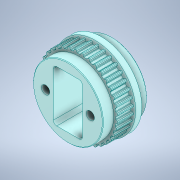
# Autodesk Inventor part: transmission_pulley_at3_t30_output
Saved by Autodesk Inventor 2022.2 (Build 262287000, 287)
## iProperties
Created: 2019-07-05
Part Number: transmission_pulley_at3_t30_output
Material: solidworks materials|PMMA
Document SubType Name: Modeling
Designer: Jochen
Density: 1.19 g/cm^3
Appearance: 192,255,255
Sending System: SolidWorks 2017
Last Author: Felix
Last Saved: 2021-02-23
Author: Jochen
Autodesk Inventor part; units mm, degrees
ref_plane "YZ Plane" through (0, 0, 0) normal (1, 0, 0) x (0, 1, 0)
ref_plane "XZ Plane" through (0, 0, 0) normal (0, 1, 0) x (-1, 0, 0)
feature "Fase1" [suppressed]
ref_plane "Work Plane1" through (0, 0, 20) normal (0, 0, 1) x (1, 0, 0)
sketch "Sketch1" plane through (0, 0, 20) normal (0, 0, 1) x (1, 0, 0)
  line L0 (-20.3, 0) -> (20.3, 0) construction
  line L1 (0, -20.3) -> (0, 20.3) construction
  line L2 (-4, -9) -> (4, -9)
  line L3 (5, -8) -> (5, 8) construction
  line L4 (4, 9) -> (-4, 9) construction
  line L5 (-5, 8) -> (-5, -8) construction
  line L6 (-5, -9) -> (5, 9) construction
  line L7 (5, -9) -> (-5, 9) construction
  circle A0 centre (0, 0) radius 12.5
  circle A1 centre (8, 0) radius 1.5
  circle A2 centre (-8, 0) radius 1.5
  arc A3 (-3.1617, 13.4663) -> (-3.482, 13.5848) centre (-3.4075, 13.2942) ccw
  arc A4 (-3.482, 13.5848) -> (-3.7769, 13.5058) centre (0, 0) ccw
  arc A5 (-3.7769, 13.5058) -> (-3.995, 13.243) centre (-3.6961, 13.2169) ccw
  line L8 (-3.995, 13.243) -> (-4.0355, 12.7799)
  arc A6 (-4.1663, 12.6094) -> (-4.0355, 12.7799) centre (-4.2348, 12.7973) ccw
  line L9 (-4.1663, 12.6094) -> (-4.9136, 12.3374)
  arc A7 (-5.1234, 12.384) -> (-4.9136, 12.3374) centre (-4.982, 12.5254) ccw
  line L10 (-5.1234, 12.384) -> (-5.4521, 12.7127)
  arc A8 (-5.4521, 12.7127) -> (-5.788, 12.7738) centre (-5.6642, 12.5005) ccw
  arc A9 (-5.788, 12.7738) -> (-6.0648, 12.6447) centre (0, 0) ccw
  arc A10 (-6.0648, 12.6447) -> (-6.2339, 12.3481) centre (-5.9351, 12.3742) ccw
  line L11 (-6.2339, 12.3481) -> (-6.1934, 11.885)
  arc A11 (-6.2927, 11.6944) -> (-6.1934, 11.885) centre (-6.3927, 11.8676) ccw
  line L12 (-6.2927, 11.6944) -> (-6.9813, 11.2968)
  arc A12 (-7.196, 11.3062) -> (-6.9813, 11.2968) centre (-7.0813, 11.47) ccw
  line L13 (-7.196, 11.3062) -> (-7.5768, 11.5728)
  arc A13 (-7.5768, 11.5728) -> (-7.9183, 11.5746) centre (-7.7489, 11.327) ccw
  arc A14 (-7.9183, 11.5746) -> (-8.1684, 11.3995) centre (0, 0) ccw
  arc A15 (-8.1684, 11.3995) -> (-8.2834, 11.078) centre (-7.9937, 11.1556) ccw
  line L14 (-8.2834, 11.078) -> (-8.1631, 10.629)
  arc A16 (-8.2278, 10.424) -> (-8.1631, 10.629) centre (-8.3563, 10.5772) ccw
  line L15 (-8.2278, 10.424) -> (-8.8369, 9.9129)
  arc A17 (-9.05, 9.8848) -> (-8.8369, 9.9129) centre (-8.9655, 10.0661) ccw
  line L16 (-9.05, 9.8848) -> (-9.4713, 10.0813)
  arc A18 (-9.4713, 10.0813) -> (-9.8079, 10.0238) centre (-9.5981, 9.8094) ccw
  arc A19 (-9.8079, 10.0238) -> (-10.0238, 9.8079) centre (0, 0) ccw
  arc A20 (-10.0238, 9.8079) -> (-10.0813, 9.4713) centre (-9.8094, 9.5981) ccw
  line L17 (-10.0813, 9.4713) -> (-9.8848, 9.05)
  arc A21 (-9.9129, 8.8369) -> (-9.8848, 9.05) centre (-10.0661, 8.9655) ccw
  line L18 (-9.9129, 8.8369) -> (-10.424, 8.2278)
  arc A22 (-10.629, 8.1631) -> (-10.424, 8.2278) centre (-10.5772, 8.3563) ccw
  line L19 (-10.629, 8.1631) -> (-11.078, 8.2834)
  arc A23 (-11.078, 8.2834) -> (-11.3995, 8.1684) centre (-11.1556, 7.9937) ccw
  arc A24 (-11.3995, 8.1684) -> (-11.5746, 7.9183) centre (0, 0) ccw
  arc A25 (-11.5746, 7.9183) -> (-11.5728, 7.5768) centre (-11.327, 7.7489) ccw
  line L20 (-11.5728, 7.5768) -> (-11.3062, 7.196)
  arc A26 (-11.2968, 6.9813) -> (-11.3062, 7.196) centre (-11.47, 7.0813) ccw
  line L21 (-11.2968, 6.9813) -> (-11.6944, 6.2927)
  arc A27 (-11.885, 6.1934) -> (-11.6944, 6.2927) centre (-11.8676, 6.3927) ccw
  line L22 (-11.885, 6.1934) -> (-12.3481, 6.2339)
  arc A28 (-12.3481, 6.2339) -> (-12.6447, 6.0648) centre (-12.3742, 5.9351) ccw
  arc A29 (-12.6447, 6.0648) -> (-12.7738, 5.788) centre (0, 0) ccw
  arc A30 (-12.7738, 5.788) -> (-12.7127, 5.4521) centre (-12.5005, 5.6642) ccw
  line L23 (-12.7127, 5.4521) -> (-12.384, 5.1234)
  arc A31 (-12.3374, 4.9136) -> (-12.384, 5.1234) centre (-12.5254, 4.982) ccw
  line L24 (-12.3374, 4.9136) -> (-12.6094, 4.1663)
  arc A32 (-12.7799, 4.0355) -> (-12.6094, 4.1663) centre (-12.7973, 4.2348) ccw
  line L25 (-12.7799, 4.0355) -> (-13.243, 3.995)
  arc A33 (-13.243, 3.995) -> (-13.5058, 3.7769) centre (-13.2169, 3.6961) ccw
  arc A34 (-13.5058, 3.7769) -> (-13.5848, 3.482) centre (0, 0) ccw
  arc A35 (-13.5848, 3.482) -> (-13.4663, 3.1617) centre (-13.2942, 3.4075) ccw
  line L26 (-13.4663, 3.1617) -> (-13.0855, 2.8951)
  arc A36 (-13.0032, 2.6965) -> (-13.0855, 2.8951) centre (-13.2002, 2.7313) ccw
  line L27 (-13.0032, 2.6965) -> (-13.1413, 1.9135)
  arc A37 (-13.2865, 1.755) -> (-13.1413, 1.9135) centre (-13.3383, 1.9482) ccw
  line L28 (-13.2865, 1.755) -> (-13.7355, 1.6347)
  arc A38 (-13.7355, 1.6347) -> (-13.9564, 1.3743) centre (-13.6579, 1.3449) ccw
  arc A39 (-13.9564, 1.3743) -> (-13.9831, 1.0701) centre (0, 0) ccw
  arc A40 (-13.9831, 1.0701) -> (-13.8107, 0.7753) centre (-13.6839, 1.0472) ccw
  line L29 (-13.8107, 0.7753) -> (-13.3894, 0.5788)
  arc A41 (-13.2739, 0.3976) -> (-13.3894, 0.5788) centre (-13.4739, 0.3976) ccw
  line L30 (-13.2739, 0.3976) -> (-13.2739, -0.3976)
  arc A42 (-13.3894, -0.5788) -> (-13.2739, -0.3976) centre (-13.4739, -0.3976) ccw
  line L31 (-13.3894, -0.5788) -> (-13.8107, -0.7753)
  arc A43 (-13.8107, -0.7753) -> (-13.9831, -1.0701) centre (-13.6839, -1.0472) ccw
  arc A44 (-13.9831, -1.0701) -> (-13.9564, -1.3743) centre (0, 0) ccw
  arc A45 (-13.9564, -1.3743) -> (-13.7355, -1.6347) centre (-13.6579, -1.3449) ccw
  line L32 (-13.7355, -1.6347) -> (-13.2865, -1.755)
  arc A46 (-13.1413, -1.9135) -> (-13.2865, -1.755) centre (-13.3383, -1.9482) ccw
  line L33 (-13.1413, -1.9135) -> (-13.0032, -2.6965)
  arc A47 (-13.0855, -2.8951) -> (-13.0032, -2.6965) centre (-13.2002, -2.7313) ccw
  line L34 (-13.0855, -2.8951) -> (-13.4663, -3.1617)
  arc A48 (-13.4663, -3.1617) -> (-13.5848, -3.482) centre (-13.2942, -3.4075) ccw
  arc A49 (-13.5848, -3.482) -> (-13.5058, -3.7769) centre (0, 0) ccw
  arc A50 (-13.5058, -3.7769) -> (-13.243, -3.995) centre (-13.2169, -3.6961) ccw
  line L35 (-13.243, -3.995) -> (-12.7799, -4.0355)
  arc A51 (-12.6094, -4.1663) -> (-12.7799, -4.0355) centre (-12.7973, -4.2348) ccw
  line L36 (-12.6094, -4.1663) -> (-12.3374, -4.9136)
  arc A52 (-12.384, -5.1234) -> (-12.3374, -4.9136) centre (-12.5254, -4.982) ccw
  line L37 (-12.384, -5.1234) -> (-12.7127, -5.4521)
  arc A53 (-12.7127, -5.4521) -> (-12.7738, -5.788) centre (-12.5005, -5.6642) ccw
  arc A54 (-12.7738, -5.788) -> (-12.6447, -6.0648) centre (0, 0) ccw
  arc A55 (-12.6447, -6.0648) -> (-12.3481, -6.2339) centre (-12.3742, -5.9351) ccw
  line L38 (-12.3481, -6.2339) -> (-11.885, -6.1934)
  arc A56 (-11.6944, -6.2927) -> (-11.885, -6.1934) centre (-11.8676, -6.3927) ccw
  line L39 (-11.6944, -6.2927) -> (-11.2968, -6.9813)
  arc A57 (-11.3062, -7.196) -> (-11.2968, -6.9813) centre (-11.47, -7.0813) ccw
  line L40 (-11.3062, -7.196) -> (-11.5728, -7.5768)
  arc A58 (-11.5728, -7.5768) -> (-11.5746, -7.9183) centre (-11.327, -7.7489) ccw
  arc A59 (-11.5746, -7.9183) -> (-11.3995, -8.1684) centre (0, 0) ccw
  arc A60 (-11.3995, -8.1684) -> (-11.078, -8.2834) centre (-11.1556, -7.9937) ccw
  line L41 (-11.078, -8.2834) -> (-10.629, -8.1631)
  arc A61 (-10.424, -8.2278) -> (-10.629, -8.1631) centre (-10.5772, -8.3563) ccw
  line L42 (-10.424, -8.2278) -> (-9.9129, -8.8369)
  arc A62 (-9.8848, -9.05) -> (-9.9129, -8.8369) centre (-10.0661, -8.9655) ccw
  line L43 (-9.8848, -9.05) -> (-10.0813, -9.4713)
  arc A63 (-10.0813, -9.4713) -> (-10.0238, -9.8079) centre (-9.8094, -9.5981) ccw
  arc A64 (-10.0238, -9.8079) -> (-9.8079, -10.0238) centre (0, 0) ccw
  arc A65 (-9.8079, -10.0238) -> (-9.4713, -10.0813) centre (-9.5981, -9.8094) ccw
  line L44 (-9.4713, -10.0813) -> (-9.05, -9.8848)
  arc A66 (-8.8369, -9.9129) -> (-9.05, -9.8848) centre (-8.9655, -10.0661) ccw
  line L45 (-8.8369, -9.9129) -> (-8.2278, -10.424)
  arc A67 (-8.1631, -10.629) -> (-8.2278, -10.424) centre (-8.3563, -10.5772) ccw
  line L46 (-8.1631, -10.629) -> (-8.2834, -11.078)
  arc A68 (-8.2834, -11.078) -> (-8.1684, -11.3995) centre (-7.9937, -11.1556) ccw
  arc A69 (-8.1684, -11.3995) -> (-7.9183, -11.5746) centre (0, 0) ccw
  arc A70 (-7.9183, -11.5746) -> (-7.5768, -11.5728) centre (-7.7489, -11.327) ccw
  line L47 (-7.5768, -11.5728) -> (-7.196, -11.3062)
  arc A71 (-6.9813, -11.2968) -> (-7.196, -11.3062) centre (-7.0813, -11.47) ccw
  line L48 (-6.9813, -11.2968) -> (-6.2927, -11.6944)
  arc A72 (-6.1934, -11.885) -> (-6.2927, -11.6944) centre (-6.3927, -11.8676) ccw
  line L49 (-6.1934, -11.885) -> (-6.2339, -12.3481)
  arc A73 (-6.2339, -12.3481) -> (-6.0648, -12.6447) centre (-5.9351, -12.3742) ccw
  arc A74 (-6.0648, -12.6447) -> (-5.788, -12.7738) centre (0, 0) ccw
  arc A75 (-5.788, -12.7738) -> (-5.4521, -12.7127) centre (-5.6642, -12.5005) ccw
  line L50 (-5.4521, -12.7127) -> (-5.1234, -12.384)
  arc A76 (-4.9136, -12.3374) -> (-5.1234, -12.384) centre (-4.982, -12.5254) ccw
  line L51 (-4.9136, -12.3374) -> (-4.1663, -12.6094)
  arc A77 (-4.0355, -12.7799) -> (-4.1663, -12.6094) centre (-4.2348, -12.7973) ccw
  line L52 (-4.0355, -12.7799) -> (-3.995, -13.243)
  arc A78 (-3.995, -13.243) -> (-3.7769, -13.5058) centre (-3.6961, -13.2169) ccw
  arc A79 (-3.7769, -13.5058) -> (-3.482, -13.5848) centre (0, 0) ccw
  arc A80 (-3.482, -13.5848) -> (-3.1617, -13.4663) centre (-3.4075, -13.2942) ccw
  line L53 (-3.1617, -13.4663) -> (-2.8951, -13.0855)
  arc A81 (-2.6965, -13.0032) -> (-2.8951, -13.0855) centre (-2.7313, -13.2002) ccw
  line L54 (-2.6965, -13.0032) -> (-1.9135, -13.1413)
  arc A82 (-1.755, -13.2865) -> (-1.9135, -13.1413) centre (-1.9482, -13.3383) ccw
  line L55 (-1.755, -13.2865) -> (-1.6347, -13.7355)
  arc A83 (-1.6347, -13.7355) -> (-1.3743, -13.9564) centre (-1.3449, -13.6579) ccw
  arc A84 (-1.3743, -13.9564) -> (-1.0701, -13.9831) centre (0, 0) ccw
  arc A85 (-1.0701, -13.9831) -> (-0.7753, -13.8107) centre (-1.0472, -13.6839) ccw
  line L56 (-0.7753, -13.8107) -> (-0.5788, -13.3894)
  arc A86 (-0.3976, -13.2739) -> (-0.5788, -13.3894) centre (-0.3976, -13.4739) ccw
  line L57 (-0.3976, -13.2739) -> (0.3976, -13.2739)
  arc A87 (0.5788, -13.3894) -> (0.3976, -13.2739) centre (0.3976, -13.4739) ccw
  line L58 (0.5788, -13.3894) -> (0.7753, -13.8107)
  arc A88 (0.7753, -13.8107) -> (1.0701, -13.9831) centre (1.0472, -13.6839) ccw
  arc A89 (1.0701, -13.9831) -> (1.3743, -13.9564) centre (0, 0) ccw
  arc A90 (1.3743, -13.9564) -> (1.6347, -13.7355) centre (1.3449, -13.6579) ccw
  line L59 (1.6347, -13.7355) -> (1.755, -13.2865)
  arc A91 (1.9135, -13.1413) -> (1.755, -13.2865) centre (1.9482, -13.3383) ccw
  line L60 (1.9135, -13.1413) -> (2.6965, -13.0032)
  arc A92 (2.8951, -13.0855) -> (2.6965, -13.0032) centre (2.7313, -13.2002) ccw
  line L61 (2.8951, -13.0855) -> (3.1617, -13.4663)
  arc A93 (3.1617, -13.4663) -> (3.482, -13.5848) centre (3.4075, -13.2942) ccw
  arc A94 (3.482, -13.5848) -> (3.7769, -13.5058) centre (0, 0) ccw
  arc A95 (3.7769, -13.5058) -> (3.995, -13.243) centre (3.6961, -13.2169) ccw
  line L62 (3.995, -13.243) -> (4.0355, -12.7799)
  arc A96 (4.1663, -12.6094) -> (4.0355, -12.7799) centre (4.2348, -12.7973) ccw
  line L63 (4.1663, -12.6094) -> (4.9136, -12.3374)
  arc A97 (5.1234, -12.384) -> (4.9136, -12.3374) centre (4.982, -12.5254) ccw
  line L64 (5.1234, -12.384) -> (5.4521, -12.7127)
  arc A98 (5.4521, -12.7127) -> (5.788, -12.7738) centre (5.6642, -12.5005) ccw
  arc A99 (5.788, -12.7738) -> (6.0648, -12.6447) centre (0, 0) ccw
  arc A100 (6.0648, -12.6447) -> (6.2339, -12.3481) centre (5.9351, -12.3742) ccw
  line L65 (6.2339, -12.3481) -> (6.1934, -11.885)
  arc A101 (6.2927, -11.6944) -> (6.1934, -11.885) centre (6.3927, -11.8676) ccw
  line L66 (6.2927, -11.6944) -> (6.9813, -11.2968)
  arc A102 (7.196, -11.3062) -> (6.9813, -11.2968) centre (7.0813, -11.47) ccw
  line L67 (7.196, -11.3062) -> (7.5768, -11.5728)
  arc A103 (7.5768, -11.5728) -> (7.9183, -11.5746) centre (7.7489, -11.327) ccw
  arc A104 (7.9183, -11.5746) -> (8.1684, -11.3995) centre (0, 0) ccw
  arc A105 (8.1684, -11.3995) -> (8.2834, -11.078) centre (7.9937, -11.1556) ccw
  line L68 (8.2834, -11.078) -> (8.1631, -10.629)
  arc A106 (8.2278, -10.424) -> (8.1631, -10.629) centre (8.3563, -10.5772) ccw
  line L69 (8.2278, -10.424) -> (8.8369, -9.9129)
  arc A107 (9.05, -9.8848) -> (8.8369, -9.9129) centre (8.9655, -10.0661) ccw
  line L70 (9.05, -9.8848) -> (9.4713, -10.0813)
  arc A108 (9.4713, -10.0813) -> (9.8079, -10.0238) centre (9.5981, -9.8094) ccw
  arc A109 (9.8079, -10.0238) -> (10.0238, -9.8079) centre (0, 0) ccw
  arc A110 (10.0238, -9.8079) -> (10.0813, -9.4713) centre (9.8094, -9.5981) ccw
  line L71 (10.0813, -9.4713) -> (9.8848, -9.05)
  arc A111 (9.9129, -8.8369) -> (9.8848, -9.05) centre (10.0661, -8.9655) ccw
  line L72 (9.9129, -8.8369) -> (10.424, -8.2278)
  arc A112 (10.629, -8.1631) -> (10.424, -8.2278) centre (10.5772, -8.3563) ccw
  line L73 (10.629, -8.1631) -> (11.078, -8.2834)
  arc A113 (11.078, -8.2834) -> (11.3995, -8.1684) centre (11.1556, -7.9937) ccw
  arc A114 (11.3995, -8.1684) -> (11.5746, -7.9183) centre (0, 0) ccw
  arc A115 (11.5746, -7.9183) -> (11.5728, -7.5768) centre (11.327, -7.7489) ccw
  line L74 (11.5728, -7.5768) -> (11.3062, -7.196)
  arc A116 (11.2968, -6.9813) -> (11.3062, -7.196) centre (11.47, -7.0813) ccw
  line L75 (11.2968, -6.9813) -> (11.6944, -6.2927)
  arc A117 (11.885, -6.1934) -> (11.6944, -6.2927) centre (11.8676, -6.3927) ccw
  line L76 (11.885, -6.1934) -> (12.3481, -6.2339)
  arc A118 (12.3481, -6.2339) -> (12.6447, -6.0648) centre (12.3742, -5.9351) ccw
  arc A119 (12.6447, -6.0648) -> (12.7738, -5.788) centre (0, 0) ccw
  arc A120 (12.7738, -5.788) -> (12.7127, -5.4521) centre (12.5005, -5.6642) ccw
  line L77 (12.7127, -5.4521) -> (12.384, -5.1234)
  arc A121 (12.3374, -4.9136) -> (12.384, -5.1234) centre (12.5254, -4.982) ccw
  line L78 (12.3374, -4.9136) -> (12.6094, -4.1663)
  arc A122 (12.7799, -4.0355) -> (12.6094, -4.1663) centre (12.7973, -4.2348) ccw
  line L79 (12.7799, -4.0355) -> (13.243, -3.995)
  arc A123 (13.243, -3.995) -> (13.5058, -3.7769) centre (13.2169, -3.6961) ccw
  arc A124 (13.5058, -3.7769) -> (13.5848, -3.482) centre (0, 0) ccw
  arc A125 (13.5848, -3.482) -> (13.4663, -3.1617) centre (13.2942, -3.4075) ccw
  line L80 (13.4663, -3.1617) -> (13.0855, -2.8951)
  arc A126 (13.0032, -2.6965) -> (13.0855, -2.8951) centre (13.2002, -2.7313) ccw
  line L81 (13.0032, -2.6965) -> (13.1413, -1.9135)
  arc A127 (13.2865, -1.755) -> (13.1413, -1.9135) centre (13.3383, -1.9482) ccw
  line L82 (13.2865, -1.755) -> (13.7355, -1.6347)
  arc A128 (13.7355, -1.6347) -> (13.9564, -1.3743) centre (13.6579, -1.3449) ccw
  arc A129 (13.9564, -1.3743) -> (13.9831, -1.0701) centre (0, 0) ccw
  arc A130 (13.9831, -1.0701) -> (13.8107, -0.7753) centre (13.6839, -1.0472) ccw
  line L83 (13.8107, -0.7753) -> (13.3894, -0.5788)
  arc A131 (13.2739, -0.3976) -> (13.3894, -0.5788) centre (13.4739, -0.3976) ccw
  line L84 (13.2739, -0.3976) -> (13.2739, 0.3976)
  arc A132 (13.3894, 0.5788) -> (13.2739, 0.3976) centre (13.4739, 0.3976) ccw
  line L85 (13.3894, 0.5788) -> (13.8107, 0.7753)
  arc A133 (13.8107, 0.7753) -> (13.9831, 1.0701) centre (13.6839, 1.0472) ccw
  arc A134 (13.9831, 1.0701) -> (13.9564, 1.3743) centre (0, 0) ccw
  arc A135 (13.9564, 1.3743) -> (13.7355, 1.6347) centre (13.6579, 1.3449) ccw
  line L86 (13.7355, 1.6347) -> (13.2865, 1.755)
  arc A136 (13.1413, 1.9135) -> (13.2865, 1.755) centre (13.3383, 1.9482) ccw
  line L87 (13.1413, 1.9135) -> (13.0032, 2.6965)
  arc A137 (13.0855, 2.8951) -> (13.0032, 2.6965) centre (13.2002, 2.7313) ccw
  line L88 (13.0855, 2.8951) -> (13.4663, 3.1617)
  arc A138 (13.4663, 3.1617) -> (13.5848, 3.482) centre (13.2942, 3.4075) ccw
  arc A139 (13.5848, 3.482) -> (13.5058, 3.7769) centre (0, 0) ccw
  arc A140 (13.5058, 3.7769) -> (13.243, 3.995) centre (13.2169, 3.6961) ccw
  line L89 (13.243, 3.995) -> (12.7799, 4.0355)
  arc A141 (12.6094, 4.1663) -> (12.7799, 4.0355) centre (12.7973, 4.2348) ccw
  line L90 (12.6094, 4.1663) -> (12.3374, 4.9136)
  arc A142 (12.384, 5.1234) -> (12.3374, 4.9136) centre (12.5254, 4.982) ccw
  line L91 (12.384, 5.1234) -> (12.7127, 5.4521)
  arc A143 (12.7127, 5.4521) -> (12.7738, 5.788) centre (12.5005, 5.6642) ccw
  arc A144 (12.7738, 5.788) -> (12.6447, 6.0648) centre (0, 0) ccw
  arc A145 (12.6447, 6.0648) -> (12.3481, 6.2339) centre (12.3742, 5.9351) ccw
  line L92 (12.3481, 6.2339) -> (11.885, 6.1934)
  arc A146 (11.6944, 6.2927) -> (11.885, 6.1934) centre (11.8676, 6.3927) ccw
  line L93 (11.6944, 6.2927) -> (11.2968, 6.9813)
  arc A147 (11.3062, 7.196) -> (11.2968, 6.9813) centre (11.47, 7.0813) ccw
  line L94 (11.3062, 7.196) -> (11.5728, 7.5768)
  arc A148 (11.5728, 7.5768) -> (11.5746, 7.9183) centre (11.327, 7.7489) ccw
  arc A149 (11.5746, 7.9183) -> (11.3995, 8.1684) centre (0, 0) ccw
  arc A150 (11.3995, 8.1684) -> (11.078, 8.2834) centre (11.1556, 7.9937) ccw
  line L95 (11.078, 8.2834) -> (10.629, 8.1631)
  arc A151 (10.424, 8.2278) -> (10.629, 8.1631) centre (10.5772, 8.3563) ccw
  line L96 (10.424, 8.2278) -> (9.9129, 8.8369)
  arc A152 (9.8848, 9.05) -> (9.9129, 8.8369) centre (10.0661, 8.9655) ccw
  line L97 (9.8848, 9.05) -> (10.0813, 9.4713)
  arc A153 (10.0813, 9.4713) -> (10.0238, 9.8079) centre (9.8094, 9.5981) ccw
  arc A154 (10.0238, 9.8079) -> (9.8079, 10.0238) centre (0, 0) ccw
  arc A155 (9.8079, 10.0238) -> (9.4713, 10.0813) centre (9.5981, 9.8094) ccw
  line L98 (9.4713, 10.0813) -> (9.05, 9.8848)
  arc A156 (8.8369, 9.9129) -> (9.05, 9.8848) centre (8.9655, 10.0661) ccw
  line L99 (8.8369, 9.9129) -> (8.2278, 10.424)
  arc A157 (8.1631, 10.629) -> (8.2278, 10.424) centre (8.3563, 10.5772) ccw
  line L100 (8.1631, 10.629) -> (8.2834, 11.078)
  arc A158 (8.2834, 11.078) -> (8.1684, 11.3995) centre (7.9937, 11.1556) ccw
  arc A159 (8.1684, 11.3995) -> (7.9183, 11.5746) centre (0, 0) ccw
  arc A160 (7.9183, 11.5746) -> (7.5768, 11.5728) centre (7.7489, 11.327) ccw
  line L101 (7.5768, 11.5728) -> (7.196, 11.3062)
  arc A161 (6.9813, 11.2968) -> (7.196, 11.3062) centre (7.0813, 11.47) ccw
  line L102 (6.9813, 11.2968) -> (6.2927, 11.6944)
  arc A162 (6.1934, 11.885) -> (6.2927, 11.6944) centre (6.3927, 11.8676) ccw
  line L103 (6.1934, 11.885) -> (6.2339, 12.3481)
  arc A163 (6.2339, 12.3481) -> (6.0648, 12.6447) centre (5.9351, 12.3742) ccw
  arc A164 (6.0648, 12.6447) -> (5.788, 12.7738) centre (0, 0) ccw
  arc A165 (5.788, 12.7738) -> (5.4521, 12.7127) centre (5.6642, 12.5005) ccw
  line L104 (5.4521, 12.7127) -> (5.1234, 12.384)
  arc A166 (4.9136, 12.3374) -> (5.1234, 12.384) centre (4.982, 12.5254) ccw
  line L105 (4.9136, 12.3374) -> (4.1663, 12.6094)
  arc A167 (4.0355, 12.7799) -> (4.1663, 12.6094) centre (4.2348, 12.7973) ccw
  line L106 (4.0355, 12.7799) -> (3.995, 13.243)
  arc A168 (3.995, 13.243) -> (3.7769, 13.5058) centre (3.6961, 13.2169) ccw
  arc A169 (3.7769, 13.5058) -> (3.482, 13.5848) centre (0, 0) ccw
  arc A170 (3.482, 13.5848) -> (3.1617, 13.4663) centre (3.4075, 13.2942) ccw
  line L107 (3.1617, 13.4663) -> (2.8951, 13.0855)
  arc A171 (2.6965, 13.0032) -> (2.8951, 13.0855) centre (2.7313, 13.2002) ccw
  line L108 (2.6965, 13.0032) -> (1.9135, 13.1413)
  arc A172 (1.755, 13.2865) -> (1.9135, 13.1413) centre (1.9482, 13.3383) ccw
  line L109 (1.755, 13.2865) -> (1.6347, 13.7355)
  arc A173 (1.6347, 13.7355) -> (1.3743, 13.9564) centre (1.3449, 13.6579) ccw
  arc A174 (1.3743, 13.9564) -> (1.0701, 13.9831) centre (0, 0) ccw
  arc A175 (1.0701, 13.9831) -> (0.7753, 13.8107) centre (1.0472, 13.6839) ccw
  line L110 (0.7753, 13.8107) -> (0.5788, 13.3894)
  arc A176 (0.3976, 13.2739) -> (0.5788, 13.3894) centre (0.3976, 13.4739) ccw
  line L111 (0.3976, 13.2739) -> (-0.3976, 13.2739)
  arc A177 (-0.5788, 13.3894) -> (-0.3976, 13.2739) centre (-0.3976, 13.4739) ccw
  line L112 (-0.5788, 13.3894) -> (-0.7753, 13.8107)
  arc A178 (-0.7753, 13.8107) -> (-1.0701, 13.9831) centre (-1.0472, 13.6839) ccw
  arc A179 (-1.0701, 13.9831) -> (-1.3743, 13.9564) centre (0, 0) ccw
  arc A180 (-1.3743, 13.9564) -> (-1.6347, 13.7355) centre (-1.3449, 13.6579) ccw
  line L113 (-1.6347, 13.7355) -> (-1.755, 13.2865)
  arc A181 (-1.9135, 13.1413) -> (-1.755, 13.2865) centre (-1.9482, 13.3383) ccw
  line L114 (-1.9135, 13.1413) -> (-2.6965, 13.0032)
  arc A182 (-2.8951, 13.0855) -> (-2.6965, 13.0032) centre (-2.7313, 13.2002) ccw
  line L115 (-2.8951, 13.0855) -> (-3.1617, 13.4663)
  circle A183 centre (0, 0) radius 14.5
  arc A184 (5, 8) -> (4, 9) centre (4, 8) ccw
  arc A185 (4, -9) -> (5, -8) centre (4, -8) ccw construction
  arc A186 (-5, -8) -> (-4, -9) centre (-4, -8) ccw construction
  arc A187 (-4, 9) -> (-5, 8) centre (-4, 8) ccw
  line L116 (-4, 9.2) -> (4, 9.2)
  arc A188 (5.2, 8) -> (4, 9.2) centre (4, 8) ccw
  line L117 (5.2, 8) -> (5.2, -8)
  arc A189 (4, -9.2) -> (5.2, -8) centre (4, -8) ccw
  line L118 (4, -9.2) -> (-4, -9.2)
  arc A190 (-5.2, -8) -> (-4, -9.2) centre (-4, -8) ccw
  line L119 (-5.2, -8) -> (-5.2, 8)
  arc A191 (-4, 9.2) -> (-5.2, 8) centre (-4, 8) ccw
  dimension "d1" = 16
  dimension "d2" = 25
  dimension "d4" = 3
  dimension "d5" = 10
  dimension "d6" = 18
  dimension "d9" = 29
  dimension "d12" = 1
  dimension "d28" = 0.2
  constraints: 376 point on circle, 236 end point, 192 centre point, 10 point on line, 8 tangent, 4 equal radius, 4 parallel, 2 coincident, 2 midpoint, 2 perpendicular, 1 horizontal, 1 symmetric about line, 7 other
  measures "d1" distance of A2.centre A1.centre
  measures "d2" diameter of A0
  measures "d4" diameter of A1
  measures "d5" distance between parallel lines of L5 L3
  measures "d6" distance between parallel lines of L2 L4
  measures "d9" diameter of A183
  measures "d12" radius of A184
  measures "d28" distance between parallel lines of L4 L116
extrude "Extrusion1" add sketch "Sketch1" along normal blind 3.85 contours A0
extrude "Extrusion2" add sketch "Sketch1" along normal blind 3 from surface at 3.85 contours A0 | L115 A182 L114 A181 L113 A180 A179 A178 L112 A177 L111 A176 L110 A175 A174 A173 L109 A172 L108 A171 L107 A170 A169 A168 L106 A167 L105 A166 L104 A165 A164 A163 L103 A162 L102 A161 L101 A160 A159 A158 L100 A157 L99 A156 L98 A155 A154 A153 L97 A152 L96 A151 L95 A150 A149 A148 L94 A147 L93 A146 L92 A145 A144 A143 L91 A142 L90 A141 L89 A140 A139 A138 L88 A137 L87 A136 L86 A135 A134 A133 L85 A132 L84 A131 L83 A130 A129 A128 L82 A127 L81 A126 L80 A125 A124 A123 L79 A122 L78 A121 L77 A120 A119 A118 L76 A117 L75 A116 L74 A115 A114 A113 L73 A112 L72 A111 L71 A110 A109 A108 L70 A107 L69 A106 L68 A105 A104 A103 L67 A102 L66 A101 L65 A100 A99 A98 L64 A97 L63 A96 L62 A95 A94 A93 L61 A92 L60 A91 L59 A90 A89 A88 L58 A87 L57 A86 L56 A85 A84 A83 L55 A82 L54 A81 L53 A80 A79 A78 L52 A77 L51 A76 L50 A75 A74 A73 L49 A72 L48 A71 L47 A70 A69 A68 L46 A67 L45 A66 L44 A65 A64 A63 L43 A62 L42 A61 L41 A60 A59 A58 L40 A57 L39 A56 L38 A55 A54 A53 L37 A52 L36 A51 L35 A50 A49 A48 L34 A47 L33 A46 L32 A45 A44 A43 L31 A42 L30 A41 L29 A40 A39 A38 L28 A37 L27 A36 L26 A35 A34 A33 L25 A32 L24 A31 L23 A30 A29 A28 L22 A27 L21 A26 L20 A25 A24 A23 L19 A22 L18 A21 L17 A20 A19 A18 L16 A17 L15 A16 L14 A15 A14 A13 L13 A12 L12 A11 L11 A10 A9 A8 L10 A7 L9 A6 L8 A5 A4 A3 | A183
chamfer "Chamfer1" distance 0.8 distance2 2 1 edges at (-14.5, 0, 26.85) measured on face at (-14.5, 0, 26.35)
extrude "Extrusion3" add sketch "Sketch1" along normal blind 8.1 from surface at 3.85 contours A0 | L115 A182 L114 A181 L113 A180 A179 A178 L112 A177 L111 A176 L110 A175 A174 A173 L109 A172 L108 A171 L107 A170 A169 A168 L106 A167 L105 A166 L104 A165 A164 A163 L103 A162 L102 A161 L101 A160 A159 A158 L100 A157 L99 A156 L98 A155 A154 A153 L97 A152 L96 A151 L95 A150 A149 A148 L94 A147 L93 A146 L92 A145 A144 A143 L91 A142 L90 A141 L89 A140 A139 A138 L88 A137 L87 A136 L86 A135 A134 A133 L85 A132 L84 A131 L83 A130 A129 A128 L82 A127 L81 A126 L80 A125 A124 A123 L79 A122 L78 A121 L77 A120 A119 A118 L76 A117 L75 A116 L74 A115 A114 A113 L73 A112 L72 A111 L71 A110 A109 A108 L70 A107 L69 A106 L68 A105 A104 A103 L67 A102 L66 A101 L65 A100 A99 A98 L64 A97 L63 A96 L62 A95 A94 A93 L61 A92 L60 A91 L59 A90 A89 A88 L58 A87 L57 A86 L56 A85 A84 A83 L55 A82 L54 A81 L53 A80 A79 A78 L52 A77 L51 A76 L50 A75 A74 A73 L49 A72 L48 A71 L47 A70 A69 A68 L46 A67 L45 A66 L44 A65 A64 A63 L43 A62 L42 A61 L41 A60 A59 A58 L40 A57 L39 A56 L38 A55 A54 A53 L37 A52 L36 A51 L35 A50 A49 A48 L34 A47 L33 A46 L32 A45 A44 A43 L31 A42 L30 A41 L29 A40 A39 A38 L28 A37 L27 A36 L26 A35 A34 A33 L25 A32 L24 A31 L23 A30 A29 A28 L22 A27 L21 A26 L20 A25 A24 A23 L19 A22 L18 A21 L17 A20 A19 A18 L16 A17 L15 A16 L14 A15 A14 A13 L13 A12 L12 A11 L11 A10 A9 A8 L10 A7 L9 A6 L8 A5 A4 A3
extrude "Extrusion4" add sketch "Sketch1" along normal blind 3.85 from surface at 11.95 contours A0
chamfer "Chamfer2" distance 1 angle 45 8 edges at (0, -9.2, 20) (-4.8485, -8.8485, 20) (-5.2, 0, 20) (-4.8485, 8.8485, 20) (0, 9.2, 20) (4.8485, 8.8485, 20) (5.2, 0, 20) (4.8485, -8.8485, 20)
chamfer "Chamfer3" distance 0.2 angle 45 2 edges at (-12.5, 0, 35.8) (-12.5, 0, 20)
body "Solid1"
body "Solid2"
body "Solid3"
body "Solid4"
